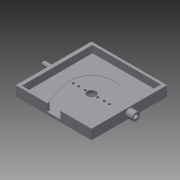
# Autodesk Inventor part: joystick_inner1
Saved by Autodesk Inventor 2015 (Build 190159000, 159)
## iProperties
Created: 2015-12-08
Part Number: joystick_inner1
Material: Generic
Document SubType Name: Modeling
Designer: boztalay
Density: 1 g/cm^3
Appearance: Default
Author: boztalay
Autodesk Inventor part; units mm, degrees
ref_plane "YZ Plane" through (0, 0, 0) normal (1, 0, 0) x (0, 1, 0)
ref_plane "XZ Plane" through (0, 0, 0) normal (0, 1, 0) x (-1, 0, 0)
ref_plane "XY Plane" through (0, 0, 0) normal (0, 0, 1) x (1, 0, 0)
sketch "Sketch1" plane through (0, 0, 0) normal (0, 1, 0) x (-1, 0, 0)
  line L0 (0, 0) -> (0, 0) construction
  line L1 (-48.26, 48.26) -> (48.26, 48.26)
  line L2 (48.26, 48.26) -> (48.26, -48.26)
  line L3 (48.26, -48.26) -> (-48.26, -48.26)
  line L4 (-48.26, -48.26) -> (-48.26, 48.26)
  line L5 (-48.26, 48.26) -> (48.26, -48.26) construction
  line L6 (48.26, 48.26) -> (-48.26, -48.26) construction
  dimension "d15" = 0
  dimension "d16" = 96.52
  constraints: 14 end point, 2 midpoint, 2 parallel, 2 perpendicular, 1 horizontal, 1 vertical
  measures "d15" distance of L0.start L0.end
  measures "d16" distance of L1.end L2.end
extrude "Extrusion2" add sketch "Sketch1" along normal blind 3.556
sketch "Sketch7" plane through (0, 3.556, 0) normal (0, 1, 0) x (1, 0, 0)
  arc A0 (27.0056, -8.0993) -> (-27.0056, -8.0993) centre (0, 0) ccw
  line L0 (0, -43.942) -> (14.366, -43.942)
  line L1 (-14.366, -43.942) -> (0, -43.942)
  line L2 (0, 15.1299) -> (0, -95.843) construction
  line L3 (33.8234, 0) -> (-34.0336, 0) construction
  line L4 (16.256, 0) -> (16.256, -43.942) construction
  line L5 (16.7989, -42.1317) -> (27.0056, -8.0993)
  line L6 (-16.7989, -42.1317) -> (-27.0056, -8.0993)
  circle A1 centre (0, 0) radius 5.5372
  arc A2 (14.366, -43.942) -> (16.7989, -42.1317) centre (14.366, -41.402) ccw
  arc A3 (-16.7989, -42.1317) -> (-14.366, -43.942) centre (-14.366, -41.402) ccw
  circle A4 centre (7.9375, 0) radius 1.524
  line L7 (0, 0) -> (7.9375, 0) construction
  circle A5 centre (-7.9375, 0) radius 1.524
  line L8 (0, 0) -> (-7.9375, 0) construction
  circle A6 centre (16.256, 0) radius 1.524
  line L9 (0, 0) -> (16.256, 0) construction
  circle A7 centre (-16.256, 0) radius 1.524
  line L10 (0, 0) -> (-16.256, 0) construction
  circle A8 centre (23.0124, 0) radius 1.524
  line L11 (0, 0) -> (23.0124, 0) construction
  circle A9 centre (-23.0124, 0) radius 1.524
  line L12 (0, 0) -> (-23.0124, 0) construction
  line L13 (-48.26, -48.26) -> (48.26, -48.26) projected
  line L14 (8.255, -39.624) -> (-8.255, -39.624)
  line L15 (-8.255, -39.624) -> (-8.255, -48.26)
  line L16 (-8.255, -48.26) -> (8.255, -48.26)
  line L17 (8.255, -48.26) -> (8.255, -39.624)
  line L18 (8.255, -39.624) -> (-8.255, -48.26) construction
  line L19 (-8.255, -39.624) -> (8.255, -48.26) construction
  point P0 (-16.256, -43.942)
  dimension "d43" = 56.388
  dimension "d44" = 16.256
  dimension "d45" = 16.256
  dimension "d46" = 43.942
  dimension "d47" = 11.0744
  dimension "d48" = 2.54
  dimension "d49" = 3.048
  dimension "d50" = 7.9375
  dimension "d51" = 3.048
  dimension "d52" = 16.256
  dimension "d53" = 3.048
  dimension "d54" = 23.0124
  dimension "d77" = 16.51
  constraints: 38 end point, 10 centre point, 10 point on line, 7 horizontal, 6 point on circle, 6 tangent, 3 symmetric about line, 3 vertical, 2 coincident, 2 collinear, 2 midpoint, 2 parallel, 1 equal radius, 1 perpendicular, 3 other
  measures "d43" diameter of A0
  measures "d44" distance of L0.start L4.end
  measures "d45" distance of L0.start point (-16.256, -43.942)
  measures "d46" distance of L4.end L4.start
  measures "d47" diameter of A1
  measures "d48" radius of A2
  measures "d49" diameter of A4
  measures "d50" distance of L7.start L7.end
  measures "d51" diameter of A6
  measures "d52" distance of L7.start L9.end
  measures "d53" diameter of A8
  measures "d54" distance of L7.start L11.end
  measures "d77" distance of L14.start L14.end
extrude "Extrusion3" cut sketch "Sketch7" against normal blind 0.381
sketch "Sketch8" plane through (0, 0, 0) normal (0, -1, 0) x (1, 0, 0)
  arc A0 (27.0056, -8.0993) -> (-27.0056, -8.0993) centre (0, 0) ccw
  line L0 (0, -43.942) -> (14.366, -43.942)
  line L1 (-14.366, -43.942) -> (0, -43.942)
  line L2 (0, 15.1299) -> (0, -95.843) construction
  line L3 (33.8234, 0) -> (-34.0336, 0) construction
  line L4 (16.256, 0) -> (16.256, -43.942) construction
  line L5 (16.7989, -42.1317) -> (27.0056, -8.0993)
  line L6 (-16.7989, -42.1317) -> (-27.0056, -8.0993)
  circle A1 centre (0, 0) radius 5.5372
  arc A2 (14.366, -43.942) -> (16.7989, -42.1317) centre (14.366, -41.402) ccw
  arc A3 (-16.7989, -42.1317) -> (-14.366, -43.942) centre (-14.366, -41.402) ccw
  circle A4 centre (7.9375, 0) radius 1.524
  line L7 (0, 0) -> (7.9375, 0) construction
  circle A5 centre (-7.9375, 0) radius 1.524
  line L8 (0, 0) -> (-7.9375, 0) construction
  circle A6 centre (16.256, 0) radius 1.524
  line L9 (0, 0) -> (16.256, 0) construction
  circle A7 centre (-16.256, 0) radius 1.524
  line L10 (0, 0) -> (-16.256, 0) construction
  circle A8 centre (23.0124, 0) radius 1.524
  line L11 (0, 0) -> (23.0124, 0) construction
  circle A9 centre (-23.0124, 0) radius 1.524
  line L12 (0, 0) -> (-23.0124, 0) construction
  point P0 (-16.256, -43.942)
  dimension "d57" = 56.388
  dimension "d58" = 16.256
  dimension "d59" = 16.256
  dimension "d60" = 43.942
  dimension "d61" = 11.0744
  dimension "d62" = 2.54
  dimension "d63" = 3.048
  dimension "d64" = 7.9375
  dimension "d65" = 3.048
  dimension "d66" = 16.256
  dimension "d67" = 3.048
  dimension "d68" = 23.0124
  constraints: 26 end point, 10 centre point, 9 point on line, 6 horizontal, 6 point on circle, 6 tangent, 3 symmetric about line, 3 vertical, 2 coincident, 2 collinear, 1 equal radius, 3 other
  measures "d57" diameter of A0
  measures "d58" distance of L0.start L4.end
  measures "d59" distance of L0.start point (-16.256, -43.942)
  measures "d60" distance of L4.end L4.start
  measures "d61" diameter of A1
  measures "d62" radius of A2
  measures "d63" diameter of A4
  measures "d64" distance of L7.start L7.end
  measures "d65" diameter of A6
  measures "d66" distance of L7.start L9.end
  measures "d67" diameter of A8
  measures "d68" distance of L7.start L11.end
extrude "Extrusion4" cut sketch "Sketch8" against normal blind 3.556 contours A1 | A4 | A5 | A6 | A7 | A8 | A9
sketch "Sketch9" plane through (0, 3.556, 0) normal (0, 1, 0) x (1, 0, 0)
  line L0 (43.815, -45.085) -> (-43.815, -45.085)
  line L1 (-43.815, -45.085) -> (-43.815, 45.085)
  line L2 (-43.815, 45.085) -> (43.815, 45.085)
  line L3 (43.815, 45.085) -> (43.815, -45.085)
  line L4 (43.815, -45.085) -> (-43.815, 45.085) construction
  line L5 (-43.815, -45.085) -> (43.815, 45.085) construction
  line L6 (48.26, -48.26) -> (-48.26, -48.26)
  line L7 (-48.26, -48.26) -> (-48.26, 48.26)
  line L8 (-48.26, 48.26) -> (48.26, 48.26)
  line L9 (48.26, 48.26) -> (48.26, -48.26)
  line L10 (48.26, -48.26) -> (-48.26, 48.26) construction
  line L11 (-48.26, -48.26) -> (48.26, 48.26) construction
  point P0 (0, 0)
  dimension "d71" = 90.17
  dimension "d72" = 87.63
  constraints: 24 end point, 4 midpoint, 4 parallel, 2 horizontal, 2 perpendicular
  measures "d71" distance of L0.end L1.end
  measures "d72" distance of L1.end L2.end
extrude "Extrusion5" add sketch "Sketch9" along normal blind 9.144
sketch "Sketch10" plane through (43.815, 3.556, 45.085) normal (0, 0, -1) x (-1, 0, 0)
  line L0 (0, 9.144) -> (87.63, 9.144) projected
  line L1 (35.5652, 0) -> (52.0648, 0)
  line L2 (52.0648, 0) -> (52.0648, 9.144)
  line L3 (52.0648, 9.144) -> (35.5652, 9.144)
  line L4 (35.5652, 9.144) -> (35.5652, 0)
  line L5 (35.5652, 0) -> (52.0648, 9.144) construction
  line L6 (52.0648, 0) -> (35.5652, 9.144) construction
  line L7 (43.815, 4.572) -> (87.63, 4.572) construction
  line L8 (43.815, 4.572) -> (0, 4.572) construction
  line L9 (0, 0) -> (0, 9.144) construction
  point P0 (43.815, -3.556)
  dimension "d88" = 28.995
  dimension "d89" = 52.0648
  constraints: 16 end point, 3 midpoint, 3 parallel, 2 horizontal, 1 collinear, 1 perpendicular, 1 point on line
  measures "d88" angle of L5 L0
  measures "d89" distance between parallel lines of L2 L9
extrude "Extrusion6" cut sketch "Sketch10" against normal up to next
sketch "Sketch14" plane through (-48.26, 0, -48.26) normal (-1, 0, 0) x (0, 0, 1)
  circle A0 centre (48.26, 6.35) radius 2.794
  line L0 (48.26, 6.35) -> (96.52, 6.35) construction
  line L1 (48.26, 6.35) -> (0, 6.35) construction
  line L2 (0, 0) -> (0, 12.7) construction
  point P0 (48.26, 0)
  dimension "d78" = 5.588
  dimension "d90" = 96.52
  constraints: 4 end point, 2 horizontal, 1 centre point, 1 collinear, 1 midpoint
  measures "d78" diameter of A0
  measures "d90" distance from line of L0.end L2
extrude "Extrusion7" add sketch "Sketch14" along normal blind 10.795
sketch "Sketch15" plane through (48.26, 0, 48.26) normal (1, 0, 0) x (0, 0, -1)
  arc A0 (50.9865, 4.7231) -> (45.5335, 4.7231) centre (48.26, 6.35) ccw
  circle A1 centre (48.26, 6.35) radius 5.08
  line L0 (45.5335, 4.7231) -> (50.9865, 4.7231)
  line L1 (48.26, 6.35) -> (0, 6.35) construction
  line L2 (0, 0) -> (0, 12.7) construction
  line L3 (48.26, 6.35) -> (96.52, 6.35) construction
  line L4 (96.52, 0) -> (96.52, 12.7) construction
  dimension "d81" = 6.35
  dimension "d82" = 10.16
  dimension "d91" = 1.6269
  constraints: 6 end point, 2 centre point, 2 midpoint, 2 point on circle, 1 coincident, 1 collinear, 1 horizontal, 1 parallel
  measures "d81" diameter of A0
  measures "d82" diameter of A1
  measures "d91" distance between parallel lines of L0 L3
extrude "Extrusion9" add sketch "Sketch15" along normal blind 6.985
body "Solid2"
